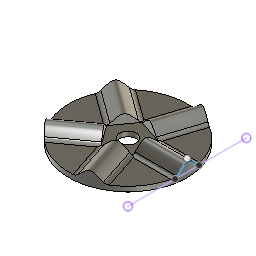
disc_up_down (Autodesk Fusion 360 design; units mm, degrees)
part number: 2026-05-12-14-40-25-549
Autodesk Fusion 360 part; units mm, degrees
sketch "disc" plane through (0, 0, 0) normal (0, 0, 1) x (1, 0, 0)
  circle A0 centre (0, 0) radius 49.5
  circle A1 centre (0, 0) radius 61.1953
  dimension "d4" = 99
  constraint coincident A0.centre A1.centre
  constraint concentric A0 A1
  measures "d4" diameter of A0
extrude "Extrude2" add sketch "disc" along normal blind 4 contours A0
ref_plane "WorkPlane1" through (49.5, 0, 2.7519) normal (1, 0, 0) x (0, -1, 0)
sketch "wave" plane through (49.5, 0, 0) normal (1, 0, 0) x (0, 1, 0)
  line L0 (49.5, 4) -> (-49.5, 4)
  spline S0 degree 2 poles (9.9609, 4) (0, 14) (-10.0579, 4) knots 0 0 0 2.501502 2.501502 2.501502 weights 1 3 1
  constraint coincident L0 S0.end
  constraint coincident L0 S0.start
extrude "Extrude3" add sketch "wave" against normal blind 35
pattern_circular "C-Pattern1" count 5 over 360 about axis through (0, 0, -11.25) along (0, 0, 1) of "Extrude3"
extrude "Extrude4" cut sketch "disc" along normal blind 30
fillet "Fillet1" radius 5 1 edges at (-19.6241, -26.57, 4)
fillet "Fillet1" radius 5 9 edges at (-31.3827, -10.3687, 4) (-31.3338, 10.453, 4) (-19.559, 26.6426, 4) (0.2588, 33.0304, 4) (19.2946, 26.8347, 4) (31.4937, 9.9609, 4) (31.4837, -10.0579, 4) (19.2054, -26.8742, 4) (0.1634, -33.0508, 4)
sketch "center" plane through (0, 0, 4) normal (0, 0, 1) x (-1, 0, 0)
  line L0 (5.5385, 17.0458) -> (-14.5, 10.5349)
  line L1 (-14.5, 10.5349) -> (-14.5, -10.5349)
  line L2 (-14.5, -10.5349) -> (5.5385, -17.0458)
  line L3 (5.5385, -17.0458) -> (17.923, 0)
  line L4 (17.923, 0) -> (5.5385, 17.0458)
  circle A0 centre (0, 0) radius 7
  constraint coincident A0.centre origin
extrude "Extrude6" cut sketch "center" against normal blind 8 contours A0
sketch "hole" plane through (0, 0, 0) normal (0, 0, 1) x (1, 0, 0)
  circle A0 centre (-25, 25) radius 4.25
  circle A1 centre (25, -25) radius 4.25
  line L0 (-25, 25) -> (25, -25)
  circle A2 centre (25, -25) radius 6
  circle A3 centre (-25, 25) radius 6
  dimension "d24" = 8.5
  dimension "d25" = 8.5
  dimension "d26" = 12
  dimension "d27" = 12
  constraint coincident A0.centre L0.start
  constraint coincident A1.centre L0.end
  constraint concentric A1 A2
  constraint concentric A0 A3
  measures "d24" diameter of A0
  measures "d25" diameter of A1
  measures "d26" diameter of A2
  measures "d27" diameter of A3
extrude "Extrude7" add sketch "hole" against normal blind 6
extrude "Extrude5" [suppressed]
sketch "Sketch1" plane through (0, 0, 0) normal (1, 0, 0) x (0, 1, 0)
  circle A0 centre (0, 30) radius 25
  dimension "d1" = 50
  measures "d1" diameter of A0
extrude "Extrude1" [suppressed]
sketch "Sketch2" plane through (0, 0, 0) normal (1, 0, 0) x (0, 1, 0)
  line L0 (130, 170) -> (140.9808, 210.9808)
  line L1 (140.9808, 210.9808) -> (110.9808, 240.9808)
  line L2 (110.9808, 240.9808) -> (70, 230)
  line L3 (70, 230) -> (59.0192, 189.0192)
  line L4 (59.0192, 189.0192) -> (89.0192, 159.0192)
  line L5 (89.0192, 159.0192) -> (130, 170)
  point P0 (100, 200)
named bodies: "disc"
